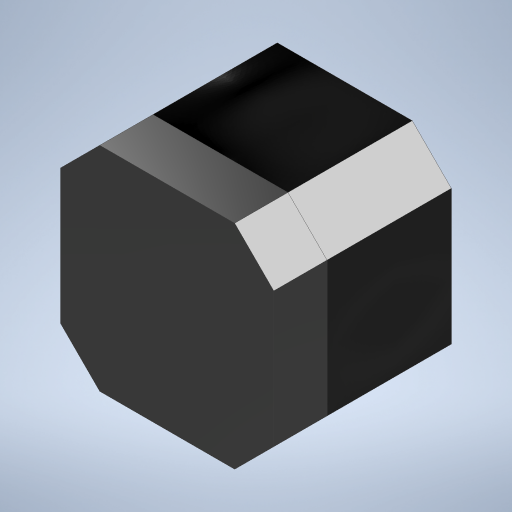
# Autodesk Inventor part: Кнопка маленькая
Saved by Autodesk Inventor 2024 (Build 280153020, 153B)
## iProperties
Created: 2022-06-07
Part Number: Кнопка маленькая
Material: Типовые
Document SubType Name: Modeling
Designer: Admin
Density: 1 g/cm^3
Appearance: По умолчанию
Author: Admin
Autodesk Inventor part; units mm, degrees
ref_plane "YZ Plane" through (0, 0, 0) normal (1, 0, 0) x (0, 1, 0)
ref_plane "XZ Plane" through (0, 0, 0) normal (0, 1, 0) x (-1, 0, 0)
ref_plane "XY Plane" through (0, 0, 0) normal (0, 0, 1) x (1, 0, 0)
sketch "Эскиз1" plane through (0, 0, 0) normal (0, 0, 1) x (1, 0, 0)
  line L0 (-3, -3) -> (3, -3)
  line L1 (3, -3) -> (3, 3)
  line L2 (3, 3) -> (-3, 3)
  line L3 (-3, 3) -> (-3, -3)
  line L4 (-3, -3) -> (3, 3) construction
  line L5 (3, -3) -> (-3, 3) construction
  line L6 (-3, 1.9) -> (-1.9, 3)
  line L7 (1.9, 3) -> (3, 1.9)
  line L8 (-3, -1.9) -> (-1.9, -3)
  line L9 (1.9, -3) -> (3, -1.9)
  point P0 (0, 0)
  dimension "d0" = 6
  dimension "d1" = 6
  dimension "d6" = 3.8
  dimension "d7" = 3.8
  constraints: 20 end point, 8 point on line, 7 perpendicular, 2 midpoint, 2 parallel, 1 horizontal
  measures "d0" distance of L2.end L1.end
  measures "d1" distance of L1.end L0.end
  measures "d6" distance of L6.end L7.start
  measures "d7" distance of L9.end L7.end
extrude "Выдавливание1" add sketch "Эскиз1" along normal blind 3.5 contours L8 L3 L6 L2 L7 L1 L9 L0
sketch "Эскиз2" plane through (0, 0, 3.5) normal (0, 0, 1) x (1, 0, 0)
  line L0 (3, -1.9) -> (3, 1.9) projected
  line L1 (1.9, 3) -> (-1.9, 3) projected
  line L2 (-3, 1.9) -> (-3, -1.9) projected
  line L3 (-1.9, -3) -> (1.9, -3) projected
  line L4 (3, 1.9) -> (1.9, 3) projected
  line L5 (-1.9, 3) -> (-3, 1.9) projected
  line L6 (-3, -1.9) -> (-1.9, -3) projected
  line L7 (1.9, -3) -> (3, -1.9) projected
  point P0 (0, 0)
extrude "Выдавливание2" add sketch "Эскиз2" along normal blind 1.5 separate body
